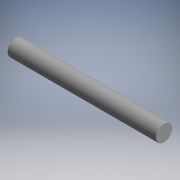
# Autodesk Inventor part: SSFHR50-450_s
Saved by Autodesk Inventor 2017.3 (Build 213256000, 256)
## iProperties
Part Number: SSFHR50-450_s
Material: Generic
Catalog Web Link: www.cadenas.de
Description: NSFMR, SFMR, PSFMR, SSFMR, NSFHR, SFHR, PSFHR, SSFHR, NSFR, SFR, PSFR, SSFR, HFR, PHFR_shaft-Rotary Shafts - Straight -
Vendor: MISUMI
Document SubType Name: Modeling
Designer: partserver
Manufacturer: MISUMI
Mass: 883.534 g
Surface Area: 745.202 cm^2
Volume: 883.534 cm^3
Density: 1 g/cm^3
Appearance: PSOLRGB-192-192-192
Category: PARTsolutions
Company: MISUMI
Title: SSFHR50-450
Author: Cadenas PARTsolutions
Comments: Rotary Shafts - Straight -
PSOL_IDENT_0: {$CADENAS_DATA\23d-libs\misumi\metric\11_rotary_shafts\11_components\psfr\psfr.prj},463 {VTYP=3D},{N
PSOL_IDENT_1: B=SSFHR50-450_s},{LINA=SSFHR50-450},{NN=NSFMR, SFMR, PSFMR, SSFMR, NSFHR, SFHR, PSFHR, SSFHR, NSFR,
PSOL_IDENT_2: SFR, PSFR, SSFR, HFR, PHFR_shaft},{DATE=05.02.2021 07:23:52},{GEOMDATE=05.02.2021 07:23:42},{VERSION=
PSOL_IDENT_3: },{LINEID=200},{WBVAR=TS,MAT,ST,ALT1,L,ALT2,KC,A,WKC,C,K,E,KZ,Z,ALT3,FC,GALT3,WFC,J,WALT3,V,ALT4,SFC
PSOL_IDENT_4: ,SG,AG,ALT10,KWC,ALT11,WC,ALT6,TA,TB,ALT5,UC,ALT7,SC,ALT32,CD},{WBNUMERIC=L,KC,A,WKC,C,K,E,KZ,Z,FC,G
PSOL_IDENT_5: ALT3,WFC,J,WALT3,V,SFC,SG,AG,KWC,WC,TA,TB,UC,SC}  {NB=SSFHR50-450_s},{LINA=SSFHR50-450},{KT=DUMMY},{
PSOL_IDENT_6: PN=SSFHR50-450},{TYPE=SSFHR},{TS=H},{TSALG= 'M','h9 (Cold-drawn)','H','h7 (Ground)','','g6 (Ground)'
PSOL_IDENT_7: },{MAT=SUS304},{MATALG= 'S45C','S45C Equivalent', 'SUS304','SUS304' },{ST=-},{STALG= '-','-' },{D=5
PSOL_IDENT_8: 0.0},{ALT1=},{L=450.0},{LALG=[100:1000/0.1]},{LMIN=100},{LMAX=1000},{ALT2=},{ALT2ALG= '', 'w/o Key G
PSOL_IDENT_9: rooves','KC','with KC (Key Groove)','WKC','with WKC (Two Key Grooves)','KCWKC','with KC + WKC (Three
PSOL_IDENT_10: Key Grooves)','KZ','with KC + WKC + KZ (Four Key Grooves)' },{ALT2PN=},{KC=0.0},{KCALG=[0]},{KCMIN=
PSOL_IDENT_11: 0},{KCMAX=0},{A=0.0},{AALG=[0]},{AMIN=14},{AMAX=0},{WKC=0.0},{WKCALG=[0]},{WKCMIN=0},{WKCMAX=0},{C=0
PSOL_IDENT_12: .0},{CALG=[0]},{CMIN=14},{CMAX=0},{K=0.0},{KALG=[0]},{KMIN=0},{KMAX=434},{E=0.0},{EALG=[0]},{EMIN=14
PSOL_IDENT_13: },{EMAX=100},{KZ=0.0},{KZALG=[0]},{KZMIN=452},{KZMAX=436},{Z=0.0},{ZALG=[0]},{ZMIN=14},{ZMAX=100},{C
PSOL_IDENT_14: IFKC=1},{CIFWKC=1},{CIFK=1},{CIFKZ=2},{PCUT3D=0.000},{QCUT3D=0},{BB=14},{BBALT2=14},{TT=5.5},{TTALT2=
PSOL_IDENT_15: 5.5},{ALT3=},{ALT3ALG= '', 'w/o Set Screw Flat','FC','with FC (Adds a Set Screw Flat)','WFC','with W
PSOL_IDENT_16: FC (Adds Two Set Screw Flats)','FCWFC','with FC + WFC (Adds Three Set Screw Flats)' },{ALT3PN=},{FC=
PSOL_IDENT_17: 0},{FCALG=[0]},{FCMIN=0},{FCMAX=449},{GALT3=0},{GALT3ALG=[0]},{GALT3MIN=1},{GALT3MAX=70},{GALT3MAX2=
PSOL_IDENT_18: 70},{GALT3MAX3=70},{WFC=0},{WFCALG=[0]},{WFCMIN=0},{WFCMIN2=2},{WFCMAX=446},{WFCMAX2=-3},{WFCMAX3=-4
PSOL_IDENT_19: },{J=0},{JALG=[0]},{JMIN=1},{JMAX=70},{JMAX2=-2},{JMAX3=-5},{WALT3=0},{WALT3ALG=[0]},{WALT3MIN=0},{W
PSOL_IDENT_20: ALT3MIN2=452},{WALT3MAX=447},{WALT3MAX2=447},{WALT3MAX3=447},{V=0},{VALG=[0]},{VMIN=1},{VMAX=70},{VM
PSOL_IDENT_21: AX2=70},{VMAX3=50},{CIFFC=0},{ALT4=},{ALT4ALG= '', 'w/o SFC (2 Set Screw Flats (Angle Specified))', '
PSOL_IDENT_22: SFC'  , 'with SFC (2 Set Screw Flats (Angle Specified))'},{ALT4PN=},{SFC=0},{SFCALG=[0]},{SFCMIN=0},
PSOL_IDENT_23: {SFCMAX=449},{SG=0},{SGALG=[0]},{SGMIN=1},{SGMAX=70},{AG=0},{AGALG=[0]},{H=0.0},{CIFSFC=0},{ALT10=},
PSOL_IDENT_24: {ALT10ALG= '', 'w/o KWC (2 Set Screw Flats at both ends)', 'KWC', 'with KWC (2 Set Screw Flats at bo
PSOL_IDENT_25: th ends)' },{ALT10PN=},{KWC=0},{KWCALG=[0]},{KWCMIN=1},{KWCMAX=224},{WALT10=45},{ALT11=},{ALT11ALG= ''
PSOL_IDENT_26: ,'Not applicable' },{ALT11PN=},{WC=0.0},{WCALG=[0]},{ALT6=},{ALT6ALG= '','w/o Retaining Ring Groove'
PSOL_IDENT_27: ,'TA','with TA (Retaining Ring Groove)','TB','with TB (Retaining Ring Groove)','TATB','with TA + TB
PSOL_IDENT_28: (Two Retaining Ring Grooves)' },{ALT6PN=},{TA=0.0},{TAALG=[0]},{TAMIN=2},{TAMAX=0},{TB=0.0},{TBALG=[
PSOL_IDENT_29: 0]},{TBMIN=2},{TBMAX=0},{DDALT6=0.0},{MM=0.00},{ALT5=},{ALT5ALG= '','Not applicable' },{ALT5PN=},{UC=
PSOL_IDENT_30: 0},{UCALG=[0]},{UCMIN=1},{UCMAX=444},{DDALT5=0},{LL1=0},{ALT7=},{ALT7ALG= '', 'w/o SC (Wrench Flats)'
PSOL_IDENT_31: , 'SC', 'with SC (Wrench Flats)'},{ALT7PN=},{SC=0},{SCALG=[0]},{SCMIN=0},{SCMAX=430},{WALT7=0},{LL2=
PSOL_IDENT_32: 0},{LL2ALG=20},{CIFSC=0},{ALT32=},{ALT32ALG=  '','w/o CD (Changes Part D Chamfering)','-CD', 'with C
PSOL_IDENT_33: D (Changes Part D Chamfering)' },{ALT32PN=},{CD=},{CDALG= '','N/A' },{CD3D=0.5},{CIF32=0},{CIF320=0}
PSOL_IDENT_34: ,{CIFTA=0},{CIFTB=0},{ERRORPN=},{ERRORALT23=OK},{ERRORALT24=OK},{ERRORALT25=OK},{ERRORALT26=OK},{ERR
PSOL_IDENT_35: ORALT27=OK},{ERRORALT210=OK},{ERRORALT34=OK},{ERRORALT35=OK},{ERRORALT36=OK},{ERRORALT37=OK},{ERRORA
PSOL_IDENT_36: LT310=OK},{ERRORALT45=OK},{ERRORALT46=OK},{ERRORALT47=OK},{ERRORALT410=OK},{ERRORALT56=OK},{ERRORALT
PSOL_IDENT_37: 57=OK},{ERRORALT510=OK},{ERRORALT610=OK},{ERRORALT75=OK},{ERRORALT76=OK},{ERRORALT710=OK}
NB: SSFHR50-450_s
NN: NSFMR, SFMR, PSFMR, SSFMR, NSFHR, SFHR, PSFHR, SSFHR, NSFR, SFR, PSFR, SSFR, HFR, PHFR_shaft
NT: Rotary Shafts - Straight -
NBSYN: $PN._s
LINA: SSFHR50-450
CATALOG: Misumi
PN: SSFHR50-450
TS: h7 (Ground)
MAT: SUS304
ST: -
D: 50
ALT1: w/o LKC (Changes L Tolerance)
L: 450
ALT2: w/o Key Grooves
KC: 0
A: 0
WKC: 0
C: 0
K: 0
E: 0
KZ: 0
Z: 0
ALT3: w/o Set Screw Flat
FC: 0
GALT3: 0
WFC: 0
J: 0
WALT3: 0
V: 0
ALT4: w/o SFC (2 Set Screw Flats (Angle Specified))
SFC: 0
SG: 0
AG: 0
H: 0
ALT10: w/o KWC (2 Set Screw Flats at both ends)
KWC: 0
ALT11: Not applicable
WC: 0
ALT6: w/o Retaining Ring Groove
TA: 0
TB: 0
DDALT6: 0
MM: 0
ALT5: Not applicable
UC: 0
DDALT5: 0
LL1: 0
ALT7: w/o SC (Wrench Flats)
SC: 0
WALT7: 0
LL2: 0
ALT32: w/o CD (Changes Part D Chamfering)
CD: N/A
SUPPLIER: MISUMI
ARTICLENO: SSFHR50-450_s
BOMINFO: SSFHR50-450
CREATOR: CADENAS GmbH
Autodesk Inventor part; units mm, degrees
sketch "Sketch_1" plane through (0, 0, 0) normal (0, 0, 1) x (1, 0, 0)
  line L0 (450, 0) -> (0, 0)
  line L1 (0, 0) -> (0, 24.5)
  line L2 (0, 24.5) -> (0.5, 25)
  line L3 (0.5, 25) -> (449.5, 25)
  line L4 (449.5, 25) -> (450, 24.5)
  line L5 (450, 24.5) -> (450, 0)
  line L6 (450, 0) -> (0, 0)
  constraints: 14 end point
revolve "Revolution1" add sketch "Sketch_1" angle 360 about axis through (450, 0, 0) along (1, 0, 0)
ref_plane "COMBINATION_MODULE_XY" through (0, 0, 0) normal (1, 0, 0) x (0, 0, -1)
ref_plane "COMBINATION_MODULE_YZ" through (0, 0, 0) normal (0, 0, -1) x (0, 1, 0)
ref_plane "COMBINATION_MODULE_ZX" through (0, 0, 0) normal (0, 1, 0) x (1, 0, 0)
body "Solid1"
